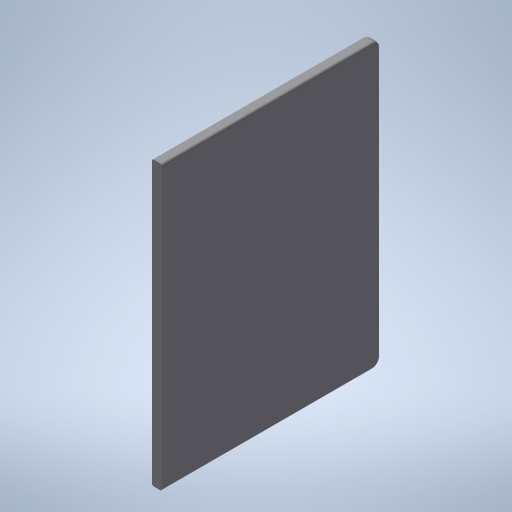
# Autodesk Inventor part: tapa de caja de servomotores
Saved by Autodesk Inventor 2023 (Build 270158000, 158)
## iProperties
Created: 2022-11-22
Part Number: tapa de caja de servomotores
Material: Generic
Document SubType Name: Modeling
Designer: Xiaba
Density: 1 g/cm^3
Appearance: Default
Author: Xiaba
Autodesk Inventor part; units mm, degrees
ref_plane "YZ Plane" through (0, 0, 0) normal (1, 0, 0) x (0, 1, 0)
ref_plane "XZ Plane" through (0, 0, 0) normal (0, 1, 0) x (-1, 0, 0)
ref_plane "XY Plane" through (0, 0, 0) normal (0, 0, 1) x (1, 0, 0)
sketch "Sketch1" plane through (0, 0, 0) normal (1, 0, 0) x (0, 1, 0)
  line L0 (0, 0) -> (70, 0)
  line L1 (70, 0) -> (70, -34)
  line L2 (70, -34) -> (0, -34)
  line L3 (0, -34) -> (0, 0)
  dimension "d0" = 34
  dimension "d1" = 70
  constraints: 8 end point, 2 parallel, 1 horizontal, 1 perpendicular
  measures "d0" distance of L0.end L1.end
  measures "d1" distance of L1.end L2.end
extrude "Extrusion1" add sketch "Sketch1" along normal blind 2.5
fillet "Fillet1" radius 2 2 edges at (1.25, 70, -34) (1.25, 0, -34)
fillet "Fillet2" radius 0.5 10 edges at (2.5, 69.4142, -33.4142) (2.5, 70, -16) (2.5, 0.5858, -33.4142) (2.5, 0, -16) (2.5, 35, -34) (0, 0.5858, -33.4142) (0, 35, -34) (0, 69.4142, -33.4142) (0, 70, -16) (0, 0, -16)
sketch "Sketch2" plane through (0, 0, 0) normal (-1, 0, 0) x (0, 0, 1)
  line L0 (0, 69.5) -> (0, 0.5) projected
  line L1 (7, 40) -> (-7, 40)
  line L2 (-7, 40) -> (-7, 30)
  line L3 (-7, 30) -> (7, 30)
  line L4 (7, 30) -> (7, 40)
  line L5 (0, 69.5) -> (0, 0.5) projected
  line L6 (7, 40) -> (-7, 30) construction
  line L7 (-7, 40) -> (7, 30) construction
  line L8 (-3, 40) -> (-3, 30)
  point P0 (0, 0)
  point P1 (0, 35)
  point P2 (-7, 35)
  point P3 (-3, 35)
  dimension "d6" = 10
  dimension "d7" = 14
  dimension "d8" = 4
  constraints: 14 end point, 5 midpoint, 2 parallel, 2 perpendicular, 2 point on line, 1 horizontal
  measures "d6" distance of L3.end L1.start
  measures "d7" distance of L2.end L3.end
  measures "d8" distance of point (-7, 35) point (-3, 35)
extrude "Extrusion2" add sketch "Sketch2" along normal blind 5 contours L8 L3 L2 L1
fillet "Fillet3" radius 2 4 edges at (-2.5, 40, -3) (-2.5, 30, -3) (-2.5, 30, -7) (-2.5, 40, -7)
fillet "Fillet4" radius 0.5 4 edges at (-5, 30.5856, -3.5856) (-5, 35, -3) (-5, 39.4144, -3.5856) (-5, 35, -7)
sketch "Sketch3" plane through (0, 0.5, 0) normal (0, 0, 1) x (1, 0, 0)
  arc A0 (2.5, 69) -> (2, 69.5) centre (2, 69) ccw projected
  arc A1 (0.5, 69.5) -> (0, 69) centre (0.5, 69) ccw projected
  arc A2 (0.5, 69.5) -> (0, 69) centre (0.5, 69) ccw projected
  line L0 (0, 69) -> (0, 0) projected
  arc A3 (0, 0) -> (0.5, -0.5) centre (0.5, 0) ccw projected
  line L1 (0.5, -0.5) -> (2, -0.5) projected
  arc A4 (2, -0.5) -> (2.5, 0) centre (2, 0) ccw projected
  line L2 (2.5, 69) -> (2.5, 0) projected
  arc A5 (2.5, 69) -> (2, 69.5) centre (2, 69) ccw projected
  line L3 (0.5, 69.5) -> (2, 69.5) projected
  point P0 (0, -0.5)
  point P1 (0, 69)
extrude "Extrusion3" add sketch "Sketch3" along normal blind 20
body "Solid1"
